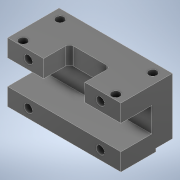
# Autodesk Inventor part: Apoio Motor
Saved by Autodesk Inventor 2021 (Build 250183000, 183)
## iProperties
Created: 2022-10-29
Part Number: Apoio Motor
Material: Plástico PC/ABS
Document SubType Name: Modeling
Designer: nicho
Density: 0.357273 g/cm^3
Appearance: Liso - Preto
Mass: 9.41358 g
Surface Area: 90.4249 cm^2
Volume: 26.3484 cm^3
Author: nicho
Autodesk Inventor part; units mm, degrees
ref_plane "YZ Plane" through (0, 0, 0) normal (1, 0, 0) x (0, 1, 0)
ref_plane "XZ Plane" through (0, 0, 0) normal (0, 1, 0) x (-1, 0, 0)
sketch "Esboço1" plane through (0, 0, 0) normal (1, 0, 0) x (0, 1, 0)
  line L0 (-17.5, 12.5) -> (17.5, 12.5)
  line L1 (17.5, 12.5) -> (17.5, -12.5)
  line L2 (17.5, -12.5) -> (-17.5, -12.5)
  line L3 (-17.5, -12.5) -> (-17.5, 12.5)
  line L4 (-17.5, 12.5) -> (17.5, -12.5) construction
  line L5 (17.5, 12.5) -> (-17.5, -12.5) construction
  point P0 (0, 0)
  dimension "d0" = 35
  dimension "d1" = 25
  constraints: 12 end point, 2 midpoint, 2 parallel, 1 horizontal, 1 perpendicular
  measures "d0" distance of L1.end L2.end
  measures "d1" distance of L0.end L1.end
extrude "Extrusão1" add sketch "Esboço1" along normal blind 55
sketch "Esboço2" plane through (0, -17.5, -12.5) normal (0, -1, 0) x (1, 0, 0)
  line L0 (55, 0) -> (55, 25) projected
  line L1 (0, 0) -> (55, 0)
  line L2 (55, 0) -> (55, 8)
  line L3 (55, 8) -> (0, 8)
  line L4 (0, 8) -> (0, 0)
  point P0 (0, 12.5)
  point P1 (55, 0)
  dimension "d4" = 8
  constraints: 8 end point, 2 parallel, 1 horizontal, 1 perpendicular, 1 point on line
  measures "d4" distance of L2.end L1.end
extrude "Extrusão2" cut sketch "Esboço2" against normal blind 1.5
sketch "Esboço3" plane through (0, 0, 0) normal (-1, 0, 0) x (0, 0, 1)
  line L0 (-2.5, 3) -> (12.5, 3)
  line L1 (12.5, 3) -> (12.5, -9)
  line L2 (12.5, -9) -> (-2.5, -9)
  line L3 (-2.5, -9) -> (-2.5, 3)
  line L4 (12.5, -17.5) -> (-4.5, -17.5) projected
  line L5 (12.5, 17.5) -> (12.5, -17.5) projected
  point P0 (0, 0)
  dimension "d7" = 15
  dimension "d8" = 12
  dimension "d9" = 8.5
  constraints: 8 end point, 2 parallel, 1 horizontal, 1 perpendicular, 1 point on line
  measures "d7" distance of L1.end L2.end
  measures "d8" distance of L0.end L1.end
  measures "d9" distance between parallel lines of L4 L2
extrude "Extrusão3" cut sketch "Esboço3" against normal through all
sketch "Esboço4" plane through (0, 0, 0) normal (-1, 0, 0) x (0, 0, 1)
  line L0 (-12.5, 17.5) -> (12.5, 17.5) projected
  line L1 (12.5, 17.5) -> (12.5, 3) projected
  line L2 (-12.5, 17.5) -> (12.5, 17.5)
  line L3 (12.5, 17.5) -> (12.5, 11.5)
  line L4 (12.5, 11.5) -> (-12.5, 11.5)
  line L5 (-12.5, 11.5) -> (-12.5, 17.5)
  line L6 (-2.5, 3) -> (12.5, 3) projected
  point P0 (0, 0)
  dimension "d12" = 8.5
  constraints: 8 end point, 2 parallel, 1 horizontal, 1 perpendicular, 1 point on line
  measures "d12" distance between parallel lines of L6 L4
extrude "Extrusão4" cut sketch "Esboço4" against normal through all
sketch "Esboço5" plane through (0, -16, -12.5) normal (0, -1, 0) x (1, 0, 0)
  line L0 (55, 8) -> (55, 0) projected
  line L1 (0, 8) -> (55, 8) projected
  line L2 (0, 0) -> (0, 8) projected
  line L3 (55, 0) -> (0, 0) projected
  point P0 (0, 12.5)
  point P1 (45, 5)
  point P2 (27.5, 5)
  point P3 (10, 5)
  dimension "d15" = 5
  dimension "d16" = 27.5
  dimension "d17" = 10
  dimension "d18" = 10
  constraints: 2 horizontal alignment
  measures "d15" distance from line of L3 point (27.5, 5)
  measures "d16" distance from line of L2 point (27.5, 5)
  measures "d17" distance from line of L2 point (10, 5)
  measures "d18" distance from line of L0 point (45, 5)
hole "Furo1" at (45, -16, -7.5) at (27.5, -16, -7.5) at (10, -16, -7.5) direction (0, 1, 0) diameter 4 depth 5
sketch "Esboço6" plane through (0, 11.5, 12.5) normal (0, 1, 0) x (1, 0, 0)
  line L0 (37.5, 12.5) -> (17.5, 12.5)
  line L1 (17.5, 12.5) -> (17.5, 0)
  line L2 (17.5, 0) -> (37.5, 0)
  line L3 (37.5, 0) -> (37.5, 12.5)
  line L4 (37.5, 12.5) -> (17.5, 0) construction
  line L5 (17.5, 12.5) -> (37.5, 0) construction
  line L6 (55, 25) -> (55, 0) projected
  line L7 (55, 0) -> (0, 0) projected
  point P0 (0, 12.5)
  point P1 (27.5, 6.25)
  dimension "d26" = 20
  dimension "d27" = 12.5
  dimension "d28" = 27.5
  constraints: 12 end point, 2 midpoint, 2 parallel, 1 horizontal, 1 perpendicular, 1 point on line
  measures "d26" distance of L2.end L1.end
  measures "d27" distance of L1.end L0.end
  measures "d28" distance from line of L6 point (27.5, 6.25)
extrude "Extrusão5" cut sketch "Esboço6" against normal up to surface (20.5 mm away)
fillet "Arredondamento1" radius 2 2 edges at (37.5, 7.25, 0) (17.5, 7.25, 0)
sketch "Esboço8" plane through (0, 11.5, 12.5) normal (0, 1, 0) x (1, 0, 0)
  line L0 (55, 0) -> (0, 0) projected
  line L1 (0, 25) -> (55, 25) projected
  line L2 (55, 25) -> (55, 0) projected
  line L3 (0, 0) -> (0, 25) projected
  line L4 (19.5, 12.5) -> (35.5, 12.5) projected
  arc A0 (37.5, 10.5) -> (35.5, 12.5) centre (35.5, 10.5) ccw projected
  line L5 (37.5, 10.5) -> (37.5, 0) projected
  line L6 (17.5, 0) -> (17.5, 10.5) projected
  arc A1 (19.5, 12.5) -> (17.5, 10.5) centre (19.5, 10.5) ccw projected
  line L7 (55, 25) -> (55, 0) projected
  line L8 (0, 25) -> (55, 25) projected
  line L9 (0, 0) -> (0, 25) projected
  line L10 (55, 0) -> (37.5, 0) projected
  line L11 (17.5, 0) -> (0, 0) projected
  point P0 (0, 12.5)
  point P1 (5, 2.5)
  point P2 (5, 20.5)
  point P3 (50, 2.5)
  point P4 (50, 20.5)
  dimension "d45" = 2.5
  dimension "d46" = 4.5
  dimension "d47" = 5
  dimension "d48" = 5
  constraints: 2 horizontal alignment, 2 vertical alignment
  measures "d45" distance from line of L0 point (5, 2.5)
  measures "d46" distance from line of L1 point (5, 20.5)
  measures "d47" distance from line of L2 point (50, 20.5)
  measures "d48" distance from line of L3 point (5, 20.5)
hole "Furo3" at (5, 11.5, 10) at (5, 11.5, -8) at (50, 11.5, 10) at (50, 11.5, -8) direction (0, -1, 0) diameter 4 depth 5
ref_plane "Plano de trabalho2" through (0, 11.5, 12.5) normal (0, 0, 1) x (1, 0, 0)
sketch "Esboço9" plane through (0, 11.5, 12.5) normal (0, 0, 1) x (1, 0, 0)
  line L0 (55, 0) -> (0, 0) projected
  line L1 (0, 0) -> (0, -8.5) projected
  line L2 (55, 0) -> (37.5, 0) projected
  line L3 (0, 0) -> (0, -8.5) projected
  line L4 (0, -8.5) -> (17.5, -8.5) projected
  line L5 (55, 0) -> (55, -8.5) projected
  line L6 (55, -20.5) -> (0, -20.5) projected
  line L7 (0, -20.5) -> (0, -29) projected
  line L8 (0, -29) -> (55, -29) projected
  line L9 (55, -20.5) -> (55, -29) projected
  line L10 (17.5, -8.5) -> (17.5, 0) projected
  line L11 (17.5, 0) -> (0, 0) projected
  line L12 (37.5, 0) -> (37.5, -8.5) projected
  line L13 (37.5, -8.5) -> (55, -8.5) projected
  point P0 (0, -11.5)
  point P1 (10, -4.25)
  point P2 (45, -24.75)
  point P3 (10, -24.75)
  point P4 (45, -4.25)
  dimension "d56" = 4.25
  dimension "d57" = 10
  dimension "d58" = 4.25
  dimension "d59" = 10
  constraints: 2 horizontal alignment, 2 vertical alignment
  measures "d56" distance from line of L0 point (10, -4.25)
  measures "d57" distance from line of L1 point (10, -4.25)
  measures "d58" distance from line of L8 point (10, -24.75)
  measures "d59" distance from line of L5 point (45, -4.25)
hole "Furo4" at (10, 7.25, 12.5) at (45, -13.25, 12.5) at (10, -13.25, 12.5) at (45, 7.25, 12.5) direction (0, 0, -1) diameter 4 depth 5
equation "\"d18\" = d17"
equation "\"d58\" = d56"
equation "\"d59\" = d57"
